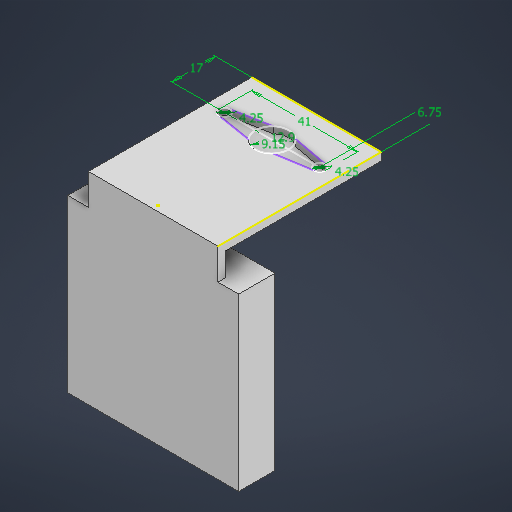
# Autodesk Inventor part: pan_base_holder_third_v2
Saved by Autodesk Inventor 2026 (Build 300175000, 175)
## iProperties
Created: 2025-06-27
Part Number: pan_base_holder_third_v2
Material: Generic
Document SubType Name: Modeling
Designer: user
Density: 1 g/cm^3
Appearance: Default
Author: user
Autodesk Inventor part; units mm, degrees
ref_plane "YZ Plane" through (0, 0, 0) normal (1, 0, 0) x (0, 1, 0)
ref_plane "XZ Plane" through (0, 0, 0) normal (0, 1, 0) x (-1, 0, 0)
ref_plane "XY Plane" through (0, 0, 0) normal (0, 0, 1) x (1, 0, 0)
sketch "Sketch1" plane through (0, 0, 0) normal (0, 0, 1) x (1, 0, 0)
  line L0 (-31, -31) -> (31, -31)
  line L1 (31, -31) -> (31, 31)
  line L2 (31, 31) -> (-31, 31)
  line L3 (-31, 31) -> (-31, -31)
  line L4 (-31, -31) -> (31, 31) construction
  line L5 (31, -31) -> (-31, 31) construction
  line L6 (-33, 33) -> (33, 33)
  line L7 (33, 33) -> (33, -33)
  line L8 (33, -33) -> (-33, -33)
  line L9 (-33, -33) -> (-33, 33)
  point P0 (0, 0)
  dimension "d0" = 62
  dimension "d1" = 62
  dimension "d2" = 2
  constraints: 20 end point, 4 parallel, 2 midpoint, 2 perpendicular, 1 horizontal, 3 other
  measures "d0" distance of L1.end L2.end
  measures "d1" distance of L0.end L1.end
  measures "d2" distance between parallel lines of L2 L6
extrude "Extrusion1" add sketch "Sketch1" along normal blind 2 contours L3 L2 L1 L0 | L6 L7 L8 L9
extrude "Extrusion2" add sketch "Sketch1" against normal blind 12
sketch "Sketch2" plane through (-33, 33, 2) normal (0, 1, 0) x (1, 0, 0)
  line L0 (8, 3) -> (58, 3)
  line L1 (58, 3) -> (58, 0)
  line L2 (58, 0) -> (8, 0)
  line L3 (8, 0) -> (8, 3)
  line L4 (0, 14) -> (0, 0) projected
  line L5 (0, 14) -> (66, 14) projected
  point P0 (33, 2)
  dimension "d7" = 50
  dimension "d8" = 3
  dimension "d9" = 8
  dimension "d10" = 11
  constraints: 8 end point, 2 parallel, 1 horizontal, 1 perpendicular
  measures "d7" distance of L1.end L2.end
  measures "d8" distance of L0.end L1.end
  measures "d9" distance between parallel lines of L4 L3
  measures "d10" distance between parallel lines of L5 L0
extrude "Extrusion3" add sketch "Sketch2" along normal blind 12
sketch "Sketch3" plane through (25, 33, -1) normal (0, 0, -1) x (-1, 0, 0)
  line L0 (50, 12) -> (0, 12) projected
  line L1 (50, 0) -> (50, 12) projected
  line L2 (0, 12) -> (50, 12)
  line L3 (50, 12) -> (50, 9)
  line L4 (50, 9) -> (0, 9)
  line L5 (0, 9) -> (0, 12)
  point P0 (25, -33)
  dimension "d13" = 3
  constraints: 8 end point, 2 parallel, 1 horizontal, 1 perpendicular, 1 point on line
  measures "d13" distance of L2.end L3.end
extrude "Extrusion4" add sketch "Sketch3" along normal blind 60
sketch "Sketch7" plane through (-33, 45, 2) normal (0, 1, 0) x (1, 0, 0)
  circle A0 centre (32.875, 46) radius 6.45
  circle A1 centre (14.5, 46) radius 2.125
  circle A2 centre (51.25, 46) radius 2.125
  line L0 (14.5, 46) -> (32.875, 46)
  line L1 (32.875, 46) -> (51.25, 46)
  line L2 (51.6412, 48.0887) -> (37.1884, 50.7955)
  line L3 (51.25, 43.875) -> (37.6436, 41.6569)
  line L4 (14.5, 43.875) -> (28.1064, 41.6569)
  line L5 (14.5, 48.125) -> (28.5616, 50.7955)
  line L6 (58, 0) -> (58, 63) projected
  line L7 (8, 63) -> (58, 63) projected
  point P0 (33, 2)
  dimension "d34" = 12.9
  dimension "d35" = 4.25
  dimension "d36" = 4.25
  dimension "d37" = 41
  dimension "d38" = 9.15
  dimension "d39" = 6.75
  dimension "d40" = 17
  constraints: 12 end point, 8 point on circle, 3 centre point, 2 collinear, 1 horizontal, 1 tangent
  measures "d34" diameter of A0
  measures "d35" diameter of A1
  measures "d36" diameter of A2
  measures "d38" distance of L3.end L2.end
  measures "d39" distance from line of L6 L1.end
  measures "d40" distance from line of L7 L0.end
extrude "Extrusion8" cut sketch "Sketch7" against normal blind 2.5
body "Solid1"
